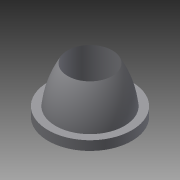
# Autodesk Inventor part: brush fitting partb v5
Saved by Autodesk Inventor 2013 SP2 (Build 170200200, 200)
## iProperties
Created: 2017-05-15
Part Number: brush fitting partb v5
Material: Generic
Document SubType Name: Modeling
Designer: Herman de Vries
Density: 1 g/cm^3
Author: Herman de Vries
Autodesk Inventor part; units mm, degrees
ref_plane "YZ Plane" through (0, 0, 0) normal (1, 0, 0) x (0, 1, 0)
ref_plane "XZ Plane" through (0, 0, 0) normal (0, 1, 0) x (-1, 0, 0)
ref_plane "XY Plane" through (0, 0, 0) normal (0, 0, 1) x (1, 0, 0)
sketch "Sketch1" plane through (0, 0, 0) normal (1, 0, 0) x (0, 1, 0)
  line L0 (0, 0) -> (7.5, 0) construction
  arc A0 (7.5, 0) -> (4.8, 10) centre (-12.3685, 0) ccw
  line L1 (0, 3.5) -> (0, 0) construction
  line L2 (4.8, 10) -> (4.8, 10)
  line L3 (7.5, 0) -> (4.8, 0)
  line L4 (4.8, 10) -> (4.8, 0)
  line L5 (4.8, 0) -> (9, 0)
  line L6 (9, 0) -> (9, 2)
  line L7 (9, 2) -> (4.8, 2)
  line L8 (4.8, 2) -> (4.8, 0)
  point P0 (0, 6.2097)
  dimension "d1" = 7.5
  dimension "d10" = 10
  dimension "d11" = 0
  dimension "d12" = 4.8
  dimension "d13" = 2
  dimension "d15" = 9
  constraints: 18 end point, 3 parallel, 2 horizontal, 2 point on circle, 2 point on line, 2 vertical, 1 centre point, 1 line through centre, 1 perpendicular
  measures "d1" distance of L0.start L0.end
  measures "d10" distance of L2.end L3.end
  measures "d11" distance of L2.start L2.end
  measures "d12" distance from line of L0.start L4
  measures "d13" distance of L5.end L6.end
  measures "d15" distance from line of L6 L0.start
revolve "Revolution1" add sketch "Sketch1" angle 360 about axis through (0, 0, 3.5) along (0, 0, -1)
body "Solid1"
